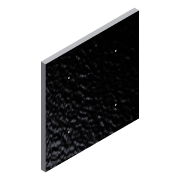
# Autodesk Inventor part: Part2
Saved by Autodesk Inventor 2013 (Build 170138000, 138)
## iProperties
Created: 2013-07-29
Part Number: Part2
Material: アルミニウム 6061
Document SubType Name: Modeling
Designer: victor
Density: 2.71 g/cm^3
Mass: 1082.64 g
Surface Area: 884.021 cm^2
Volume: 399.497 cm^3
Author: victor
Autodesk Inventor part; units mm, degrees
ref_plane "YZ Plane" through (0, 0, 0) normal (1, 0, 0) x (0, 1, 0)
ref_plane "XZ Plane" through (0, 0, 0) normal (0, 1, 0) x (-1, 0, 0)
ref_plane "XY Plane" through (0, 0, 0) normal (0, 0, 1) x (1, 0, 0)
sketch "スケッチ1" plane through (0, 0, 0) normal (1, 0, 0) x (0, 1, 0)
  line L0 (-219.8598, 80.8995) -> (-19.8598, 80.8995)
  line L1 (-19.8598, 80.8995) -> (-19.8598, -119.1005)
  line L2 (-19.8598, -119.1005) -> (-219.8598, -119.1005)
  line L3 (-219.8598, -119.1005) -> (-219.8598, 80.8995)
  point P0 (0, 0)
  dimension "d0" = 200
  dimension "d2" = 200
  constraints: 8 end point, 2 parallel, 1 horizontal, 1 perpendicular
  measures "d0" distance of L0.start L0.end
  measures "d2" distance of L0.end L1.end
extrude "押し出し1" add sketch "スケッチ1" along normal blind 10
sketch "スケッチ2" plane through (10, 0, 0) normal (1, 0, 0) x (0, 0, -1)
  line L0 (-80.8995, -19.8598) -> (-80.8995, -219.8598) projected
  line L1 (119.1005, -19.8598) -> (-80.8995, -19.8598) projected
  point P0 (0, 0)
  point P1 (-30.8995, -69.8598)
  point P2 (69.1005, -69.8598)
  point P3 (69.1005, -169.8598)
  point P4 (-30.8995, -169.8598)
  dimension "d5" = 100
  dimension "d7" = 100
  dimension "d8" = 50
  dimension "d9" = 100
  dimension "d10" = 50
  measures "d5" distance of point (69.1, -69.86) point (-30.9, -69.86)
  measures "d7" distance of point (-30.9, -69.86) point (-30.9, -169.86)
  measures "d8" distance from line of L1 point (-30.9, -69.86)
  measures "d9" distance of point (69.1, -169.86) point (69.1, -69.86)
  measures "d10" distance from line of L0 point (-30.9, -69.86)
hole "穴1" at (10, -69.8598, 30.8995) at (10, -69.8598, -69.1005) at (10, -169.8598, -69.1005) at (10, -169.8598, 30.8995) direction (-1, 0, 0) diameter 4 end through all
